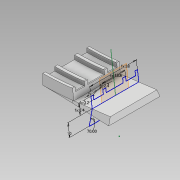
# Autodesk Inventor part: Slope_LowEnd
Saved by Autodesk Inventor 2021 (Build 250183000, 183)
## iProperties
Created: 2021-03-11
Part Number: Slope_LowEnd
Material: 一般
Document SubType Name: Modeling
Designer: kumagai
Density: 1 g/cm^3
Appearance: 既定
Author: kumagai
Autodesk Inventor part; units mm, degrees
ref_plane "YZ Plane" through (0, 0, 0) normal (1, 0, 0) x (0, 1, 0)
ref_plane "XZ Plane" through (0, 0, 0) normal (0, 1, 0) x (-1, 0, 0)
ref_plane "XY Plane" through (0, 0, 0) normal (0, 0, 1) x (1, 0, 0)
derived "SlopeProfile.ipt"
sketch "スケッチ1" plane through (0, 0, 0) normal (0, 0, 1) x (1, 0, 0)
  line L0 (0, 14) -> (0, -14)
  line L1 (-14, 0) -> (14, 0)
  line L2 (-268.75, 0) -> (268.75, 0)
  line L3 (-268.75, 0) -> (268.75, 66)
  line L4 (268.75, 66) -> (268.75, 0)
  line L5 (-31.5879, 61.457) -> (-25.6465, 13.0705)
  line L6 (-134.375, 50.6657) -> (-134.375, 8.5939)
  line L7 (23.2129, 72.7486) -> (28.7067, 28.0077)
  line L8 (-244.2356, 29.1492) -> (-240.1953, -3.7549)
  line L9 (134.375, 89.7324) -> (134.375, 45.3233)
  line L10 (239.1121, 78.5758) -> (241.9591, 55.3901)
  line L11 (-27.6764, 5.7379) -> (-27.6764, -11.9933)
  line L12 (27.6764, 6.5088) -> (27.6764, -13.0212)
  line L13 (-268.75, 0) -> (-295.625, 0)
  line L14 (268.75, 66) -> (295.625, 66)
  line L15 (241.0736, 6.6999) -> (241.0736, -9.2827)
  line L16 (-241.0736, -7.7427) -> (-241.0736, -14.414)
  arc A0 (-280.625, 0) -> (-256.9635, 1.4473) centre (-280.625, 194.1449) ccw
  line L17 (-256.3082, 4.3915) -> (-255.7778, 0.0713)
  line L18 (-280.625, 8.6126) -> (-280.625, -11.6883)
  line L19 (-295.625, 14.7784) -> (-295.625, -11.568)
  line L20 (255.3892, 69.0933) -> (256.9398, 56.465)
  line L21 (280.625, 71.1514) -> (280.625, 58.4982)
  line L22 (295.625, 71.9522) -> (295.625, 60.0478)
  arc A1 (280.625, 66) -> (256.9635, 64.5527) centre (280.625, -128.1449) ccw
  line L23 (-13.2739, 35.3851) -> (-12.039, 25.3288)
  line L24 (-43.1495, 32.5373) -> (-41.4451, 18.6566)
  line L25 (12.2235, 39.1691) -> (13.7539, 26.7059)
  line L26 (41.8424, 44.108) -> (43.6336, 29.5201)
  point P0 (0, 0)
  point P1 (-241.0736, 3.3984)
  point P2 (-27.6764, 29.6016)
  point P3 (27.6764, 36.3984)
  point P4 (241.0736, 62.6016)
  point P5 (134.375, 49.5)
  point P6 (-134.375, 16.5)
ref_plane "作業平面1" through (-241.0736, 3.3984, 0) normal (0.9925454, 0.1218753, 0) x (-0.1218753, 0.9925454, 0)
sketch "スケッチ2" plane through (-241.0736, 3.3984, 0) normal (0.9925454, 0.1218753, 0) x (-0.1218753, 0.9925454, 0)
  line L0 (-5.2, 19) -> (-5.2, -19)
  line L1 (-5.2, -19) -> (3.2, -19)
  line L2 (3.2, -19) -> (3.2, -17)
  line L3 (3.2, -17) -> (0, -17)
  line L4 (0, -17) -> (0, -9.3)
  line L5 (0, -9.3) -> (3.2, -9.3)
  line L6 (3.2, -9.3) -> (3.2, -6.9)
  line L7 (3.2, -6.9) -> (0, -6.9)
  line L8 (0, -6.9) -> (0, 6.9)
  line L9 (0, 6.9) -> (3.2, 6.9)
  line L10 (3.2, 6.9) -> (3.2, 9.3)
  line L11 (3.2, 9.3) -> (0, 9.3)
  line L12 (0, 9.3) -> (0, 17)
  line L13 (0, 17) -> (3.2, 17)
  line L14 (3.2, 17) -> (3.2, 19)
  line L15 (3.2, 19) -> (-5.2, 19)
  line L16 (25.9442, 0) -> (-7.2071, 0) projected
  line L17 (-5.2, 19) -> (-15.2, 22.6397)
  line L18 (-15.2, 22.6397) -> (-15.2, -22.6397)
  line L19 (-15.2, -22.6397) -> (-5.2, -19)
  point P0 (-32.754, 0)
  point P1 (0, 0)
  dimension "d25" = 38
  dimension "d26" = 18.6
  dimension "d27" = 2
  dimension "d28" = 2.4
  dimension "d29" = 3.2
  dimension "d30" = 8.4
  dimension "d31" = 10
  dimension "d32" = 70
  constraints: 38 end point, 10 perpendicular, 10 point on line, 2 vertical, 1 midpoint, 5 other
  measures "d25" distance between parallel lines of L1 L15
  measures "d26" distance between parallel lines of L5 L11
  measures "d27" distance between parallel lines of L15 L13
  measures "d28" distance between parallel lines of L9 L11
  measures "d29" distance between parallel lines of L12 L14
  measures "d30" distance between parallel lines of L0 L14
  measures "d31" distance between parallel lines of L18 L0
  measures "d32" angle of L17 L18
sketch "スケッチ3" plane through (0, 0, 0) normal (0, 0, 1) x (1, 0, 0)
  line L0 (-268.75, 0) -> (268.75, 66) projected
  line L1 (-241.4636, 6.5745) -> (-240.4399, -1.7628) projected
  line L2 (-256.3082, 4.3915) -> (-255.7778, 0.0713) projected
  arc A0 (-280.625, 0) -> (-256.9635, 1.4473) centre (-280.625, 194.1449) ccw projected
  line L3 (-256.9635, 1.4473) -> (-226.1855, 5.2265)
  point P0 (0, 0)
  dimension "RailWidth" = 38
  dimension "d33" = 15
  constraints: 2 end point, 1 point on line, 1 tangent
  measures "d33" distance from line of L3.end L1
sweep "スイープ1" add profiles "スケッチ2" path "スケッチ3" path curves L3 A0
extrude "押し出し1" cut sketch "スケッチ2" along normal blind 20 and the other way blind 15 contours L15 L14 L13 L12 L11 L10 L9 L8 L16 L0 | L16 L8 L7 L6 L5 L4 L3 L2 L1 L0
sketch "スケッチ4" plane through (0, 0, 0) normal (0, 0, 1) x (1, 0, 0)
  line L0 (-285.625, -5.2) -> (-220.625, -5.2)
  line L1 (-220.625, -5.2) -> (-220.625, -25.2)
  line L2 (-220.625, -25.2) -> (-285.625, -25.2)
  line L3 (-285.625, -25.2) -> (-285.625, -5.2)
  line L4 (-413.875, 0) -> (413.875, 0) projected
  line L5 (-280.625, -15.2) -> (-280.625, -5.2) projected
  point P0 (0, 0)
  dimension "RailWidth" = 38
  dimension "d40" = 5.2
  dimension "d41" = 20
  dimension "d42" = 5
  dimension "d43" = 60
  constraints: 8 end point, 3 parallel, 1 horizontal, 1 perpendicular
  measures "d40" distance between parallel lines of L0 L4
  measures "d41" distance between parallel lines of L2 L0
  measures "d42" distance between parallel lines of L5 L3
  measures "d43" distance between parallel lines of L5 L1
extrude "押し出し2" cut sketch "スケッチ4" along normal through all both and the other way through all
equation "\"d25\" = RailWidth"
equation "\"d26\" = InsideWidth"
equation "\"d27\" = OuterWall"
equation "\"d28\" = InnerWall"
equation "\"d29\" = RailDepth"
equation "\"d30\" = RailHeight"
equation "\"d37\" = ConnectorLength"
equation "\"d40\" = RailHeight - RailDepth"
equation "\"InsideWidth\" = 18.6"
equation "\"OuterWall\" = 2"
equation "\"InnerWall\" = 2.4"
equation "\"RailDepth\" = 3.2"
equation "\"RailHeight\" = 8.4"
equation "\"ConnectorLength\" = 15"
